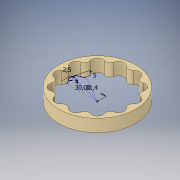
# Autodesk Inventor part: Enclosure
Saved by Autodesk Inventor 2018.3 (Build 223284000, 284)
## iProperties
Created: 2018-07-20
Part Number: Enclosure
Material: Generisch
Document SubType Name: Modeling
Designer: JochenAlt
Density: 1 g/cm^3
Appearance: Weizen
Author: JochenAlt
Autodesk Inventor part; units mm, degrees
ref_plane "YZ Plane" through (0, 0, 0) normal (1, 0, 0) x (0, 1, 0)
ref_plane "XZ Plane" through (0, 0, 0) normal (0, 1, 0) x (-1, 0, 0)
ref_plane "XY Plane" through (0, 0, 0) normal (0, 0, 1) x (1, 0, 0)
sketch "Skizze1" plane through (0, 0, 0) normal (0, 0, 1) x (1, 0, 0)
  line L0 (-46.7955, 0) -> (7.7993, 0) construction
  arc A0 (-29.3583, 16.95) -> (-33.9, 0) centre (0, 0) ccw
  arc A1 (-27.4, 0) -> (-28.7859, 3.0276) centre (-31.4, 0) ccw
  line L1 (0, 0) -> (-38.9963, 22.5145) construction
  line L2 (-31.4, 0) -> (0, 0) construction
  arc A2 (-26.4431, 11.771) -> (-23.7291, 13.7) centre (-27.1932, 15.7) ccw
  arc A3 (-30.881, 5.6855) -> (-31.4, 0) centre (0, 0) ccw construction
  arc A4 (-27.1932, 15.7) -> (-30.881, 5.6855) centre (0, 0) ccw construction
  line L3 (-37.9513, 10.169) -> (0, 0) construction
  arc A5 (-26.4431, 11.771) -> (-28.7859, 3.0276) centre (-25.5004, 6.8328) ccw
  line L4 (-23.7291, 13.7) -> (-29.3583, 16.95)
  line L5 (-27.4, 0) -> (-33.9, 0)
  point P0 (-30.3301, 8.1269)
  dimension "d5" = 4
  dimension "d14" = 31.4
  dimension "d28" = 30
  dimension "d36" = 5
  dimension "d37" = 2.5
  constraints: 15 point on circle, 10 end point, 6 centre point, 6 point on line, 2 coincident, 2 collinear, 1 equal radius, 1 tangent, 1 other
  measures "d5" radius of A1
  measures "d14" distance of L1.start L2.start
  measures "d28" angle of L1 L0
  measures "d36" distance of point (-30.33, 8.127) A5.centre
  measures "d37" radial gap between concentric circles of A0 A4
extrude "Extrusion1" add sketch "Skizze1" along normal blind 11
pattern_circular "Runde Anordnung1" count 12 over 360 about axis through (0, 0, 0) along (0, 0, 1) of "Extrusion1"
